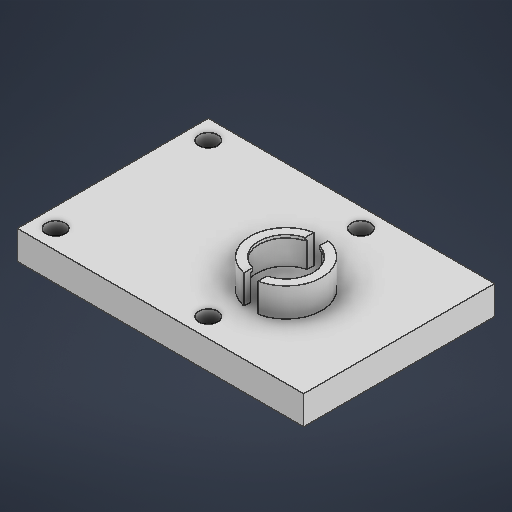
# Autodesk Inventor part: bearing_support
Saved by Autodesk Inventor 2026.1 (Build 301233000, 233)
## iProperties
Created: 2025-10-12
Part Number: bearing_support
Material: Generic
Document SubType Name: Modeling
Designer: emanuel
Density: 1 g/cm^3
Appearance: Default
Author: emanuel
Autodesk Inventor part; units mm, degrees
ref_plane "YZ Plane" through (0, 0, 0) normal (1, 0, 0) x (0, 1, 0)
ref_plane "XZ Plane" through (0, 0, 0) normal (0, 1, 0) x (-1, 0, 0)
ref_plane "XY Plane" through (0, 0, 0) normal (0, 0, 1) x (1, 0, 0)
sketch "Sketch1" plane through (0, 0, 0) normal (0, 1, 0) x (-1, 0, 0)
  line L0 (0, 0) -> (20, 0)
  line L1 (20, 0) -> (20, -20)
  line L2 (20, -20) -> (0, -20)
  line L3 (0, -20) -> (0, 0)
  line L4 (20, 0) -> (18, 0)
  line L5 (18, 0) -> (18, -2)
  line L6 (18, -2) -> (20, -2)
  line L7 (20, -2) -> (20, 0)
  line L8 (20, -20) -> (18, -20)
  line L9 (18, -20) -> (18, -18)
  line L10 (18, -18) -> (20, -18)
  line L11 (20, -18) -> (20, -20)
  line L12 (0, 0) -> (2, 0)
  line L13 (2, 0) -> (2, -2)
  line L14 (2, -2) -> (0, -2)
  line L15 (0, -2) -> (0, 0)
  line L16 (0, -20) -> (2, -20)
  line L17 (2, -20) -> (2, -18)
  line L18 (2, -18) -> (0, -18)
  line L19 (0, -18) -> (0, -20)
  circle A0 centre (2, -2) radius 1
  circle A1 centre (2, -18) radius 1
  circle A2 centre (18, -18) radius 1
  circle A3 centre (18, -2) radius 1
  line L20 (0, 0) -> (-10, 0)
  line L21 (-10, 0) -> (-10, -20)
  line L22 (-10, -20) -> (0, -20)
  line L23 (0, -20) -> (0, 0)
  dimension "d0" = 20
  dimension "d1" = 20
  dimension "d2" = 2
  dimension "d3" = 2
  dimension "d4" = 2
  dimension "d5" = 2
  dimension "d6" = 2
  dimension "d7" = 2
  dimension "d8" = 2
  dimension "d9" = 2
  dimension "d10" = 2
  dimension "d11" = 2
  dimension "d12" = 2
  dimension "d13" = 2
  dimension "d16" = 10
  constraints: 48 end point, 12 parallel, 6 horizontal, 6 perpendicular, 4 centre point, 4 coincident
  measures "d0" distance of L1.end L2.end
  measures "d1" distance of L0.end L1.end
  measures "d2" distance of L6.end L5.end
  measures "d3" distance of L5.end L4.end
  measures "d4" distance of L9.end L10.end
  measures "d5" distance of L8.end L9.end
  measures "d6" distance of L13.end L14.end
  measures "d7" distance of L12.end L13.end
  measures "d8" distance of L18.end L17.end
  measures "d9" distance of L17.end L16.end
  measures "d10" diameter of A0
  measures "d11" diameter of A1
  measures "d12" diameter of A2
  measures "d13" diameter of A3
  measures "d16" distance of L22.end L21.end
extrude "Extrusion1" add sketch "Sketch1" along normal blind 3 contours L0 L13 A0 L14 L3 | L3 L22 L21 L20 | L0 L5 A3 L6 L1 L10 A2 L9 L2 L17 A1 L18 L3 L14 A0 L13 | L0 L1 L6 A3 L5 | L18 A1 L17 L2 L3 | L1 L2 L9 A2 L10
sketch "Sketch2" plane through (0, 0, 0) normal (0, -1, 0) x (1, 0, 0)
  line L0 (-20, 0) -> (10, 0) projected
  line L1 (10, 0) -> (-0.35, 0)
  line L2 (-0.35, 0) -> (-0.35, -8.5)
  line L3 (-0.35, -8.5) -> (10, -8.5)
  line L4 (10, -8.5) -> (10, 0)
  circle A0 centre (-0.35, -8.5) radius 3.05
  circle A1 centre (-0.35, -8.5) radius 3.75
  point P0 (0, 0)
  dimension "d17" = 10.35
  dimension "d18" = 8.5
  dimension "d19" = 6.1
  dimension "d20" = 7.5
  constraints: 8 end point, 2 centre point, 2 coincident, 2 parallel, 1 horizontal, 1 perpendicular
  measures "d17" distance of L3.end L2.end
  measures "d18" distance of L2.end L1.end
  measures "d19" diameter of A0
  measures "d20" diameter of A1
extrude "Extrusion2" add sketch "Sketch2" against normal blind 6 contours A1 L3 A0 L2 | L2 A0 L3 A1
sketch "Sketch3" plane through (-0.35, 6, -8.5) normal (0, 1, 0) x (-1, 0, 0)
  circle A0 centre (0, 0) radius 3.05 projected
  circle A1 centre (0, 0) radius 3.05
  circle A2 centre (0, 0) radius 2.85
  point P0 (-0.35, 8.5)
  dimension "d23" = 5.7
  constraints: 2 centre point, 2 coincident
  measures "d23" diameter of A2
extrude "Extrusion3" add sketch "Sketch3" against normal blind 0.3
sketch "Sketch4" plane through (-0.35, 6, -8.5) normal (0, 1, 0) x (-1, 0, 0)
  line L0 (-0.75, -4.5946) -> (0.75, -4.5946)
  line L1 (0.75, -4.5946) -> (0.75, 4.5946)
  line L2 (0.75, 4.5946) -> (-0.75, 4.5946)
  line L3 (-0.75, 4.5946) -> (-0.75, -4.5946)
  circle A0 centre (0, 0) radius 2.85 projected
  line L4 (-0.75, -4.5946) -> (0.75, 4.5946) construction
  line L5 (0.75, -4.5946) -> (-0.75, 4.5946) construction
  point P0 (-0.35, 8.5)
  dimension "d26" = 1.5
  constraints: 12 end point, 2 midpoint, 2 parallel, 1 horizontal, 1 perpendicular
  measures "d26" distance of L2.end L1.end
extrude "Extrusion4" cut sketch "Sketch4" against normal blind 3 contours L3 A0 L1 L0 | L3 A0 L1 | L3 L2 L1 A0
body "Solid1"
